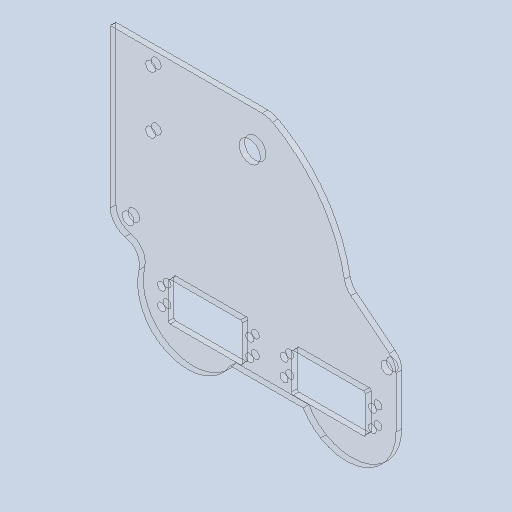
# Autodesk Inventor part: Intake Sides V4_servo
Saved by Autodesk Inventor 2022 (Build 260153000, 153)
## iProperties
Created: 2022-10-16
Part Number: Intake Sides V4_servo
Material: Polycarbonate, Clear
Document SubType Name: Modeling
Designer: matt
Density: 1.2 g/cm^3
Appearance: Polycarbonate - Clear
Mass: 60.255 g
Surface Area: 348.282 cm^2
Volume: 50.2125 cm^3
Author: matt
Autodesk Inventor part; units mm, degrees
ref_plane "YZ Plane" through (0, 0, 0) normal (1, 0, 0) x (0, 1, 0)
ref_plane "XZ Plane" through (0, 0, 0) normal (0, 1, 0) x (-1, 0, 0)
ref_plane "XY Plane" through (0, 0, 0) normal (0, 0, 1) x (1, 0, 0)
sketch "Sketch1" plane through (0, 0, 0) normal (0, 0, 1) x (1, 0, 0)
  arc A0 (16.121808, -110.692366) -> (67.383886, -131.656361) centre (43.321682, -117.338179) ccw
  line L0 (67.383886, -131.656361) -> (108.159478, -131.656361)
  arc A1 (108.159478, -131.656361) -> (139.594615, -90.326332) centre (132.221682, -117.338179) ccw
  arc A2 (132.227805, -80.679244) -> (139.594615, -90.326332) centre (142.227805, -80.679244) ccw
  line L1 (132.227805, -80.679244) -> (132.227805, -71.827)
  arc A3 (132.227805, -71.827) -> (90.658044, -1.487819) centre (51.933317, -71.827) ccw
  arc A4 (90.658044, -1.487819) -> (84.870639, 0) centre (84.870639, -12) ccw
  line L2 (84.870639, 0) -> (0, 0)
  line L3 (0, 0) -> (0, -88.644145)
  arc A5 (0, -88.644145) -> (8.203784, -98.481503) centre (10, -88.644145) ccw
  arc A6 (16.121808, -110.692366) -> (8.203784, -98.481503) centre (6.407567, -108.318861) ccw
  circle A7 centre (121.188208, -82.443861) radius 3.3
  arc A8 (145.794404, -114.286904) -> (148.095336, -110.420107) centre (146.970651, -112.368846) ccw
  circle A9 centre (97.470651, -122.368861) radius 2.25
  circle A10 centre (97.470651, -112.368852) radius 2.25
  circle A11 centre (78.175839, -122.368861) radius 2.25
  arc A12 (145.794404, -124.286918) -> (148.095336, -120.420122) centre (146.970651, -122.368861) ccw
  circle A13 centre (22.617078, -8.511936) radius 2.8
  circle A14 centre (22.617078, -40.511936) radius 2.8
  circle A15 centre (28.675839, -122.368861) radius 2.25
  circle A16 centre (28.675837, -112.368861) radius 2.25
  circle A17 centre (78.175837, -112.368855) radius 2.25
  circle A18 centre (10, -88.644145) radius 3.3
  line L4 (73.060526, -128.291526) -> (33.526976, -128.291526)
  arc A19 (32.526976, -127.291526) -> (33.526976, -128.291526) centre (33.526976, -127.291526) ccw
  line L5 (32.526976, -127.291526) -> (32.526973, -107.491526)
  arc A20 (33.526973, -106.491526) -> (32.526973, -107.491526) centre (33.526973, -107.491526) ccw
  line L6 (33.526973, -106.491526) -> (73.060526, -106.491526)
  arc A21 (74.060526, -107.491526) -> (73.060526, -106.491526) centre (73.060526, -107.491526) ccw
  line L7 (74.060526, -107.491526) -> (74.060526, -127.291526)
  arc A22 (73.060526, -128.291526) -> (74.060526, -127.291526) centre (73.060526, -127.291526) ccw
  line L8 (142.119512, -128.291526) -> (102.585962, -128.291526)
  arc A23 (101.585962, -127.291526) -> (102.585962, -128.291526) centre (102.585962, -127.291526) ccw
  line L9 (101.585962, -127.291526) -> (101.585962, -107.491526)
  arc A24 (102.585962, -106.491526) -> (101.585962, -107.491526) centre (102.585962, -107.491526) ccw
  line L10 (102.585962, -106.491526) -> (142.119515, -106.491526)
  arc A25 (143.119515, -107.491526) -> (142.119515, -106.491526) centre (142.119515, -107.491526) ccw
  line L11 (143.119515, -107.491526) -> (143.119512, -127.291526)
  arc A26 (142.119512, -128.291526) -> (143.119512, -127.291526) centre (142.119512, -127.291526) ccw
  circle A27 centre (146.970651, -112.368846) radius 2.25
  circle A28 centre (146.970651, -122.368861) radius 2.25
  line L12 (28.675837, -112.368861) -> (146.970651, -112.368846) construction
  line L13 (28.675839, -122.368861) -> (146.970651, -122.368861) construction
  circle A29 centre (43.373245, -117.368861) radius 6
  line L14 (67.43545, -131.687043) -> (108.211041, -131.687043)
  arc A30 (108.211041, -131.687043) -> (160.273251, -117.36885) centre (132.273245, -117.36885) ccw
  line L15 (160.273251, -117.36885) -> (160.273251, -88.823719)
  arc A31 (160.273251, -88.823719) -> (156.504028, -81.00212) centre (150.273251, -88.823719) ccw
  line L16 (156.504028, -81.00212) -> (134.936633, -63.821281)
  arc A32 (131.322196, -57.752321) -> (134.936633, -63.821281) centre (141.167411, -55.999682) ccw
  arc A33 (131.322196, -57.752321) -> (90.995274, -1.485865) centre (52.270547, -71.825046) ccw
  arc A34 (90.995274, -1.485865) -> (85.207869, 0.001954) centre (85.207869, -11.998046) ccw
  line L17 (85.207869, 0.001954) -> (0.051563, 0.001954)
  line L18 (0.051563, 0.001954) -> (0.051563, -88.674827)
  arc A35 (0.051563, -88.674827) -> (8.255347, -98.512185) centre (10.051563, -88.674827) ccw
  arc A36 (16.173371, -110.723048) -> (8.255347, -98.512185) centre (6.45913, -108.349543) ccw
  arc A37 (16.173371, -110.723048) -> (67.43545, -131.687043) centre (43.373245, -117.368861) ccw
  circle A38 centre (22.617078, -40.511936) radius 2.8
  circle A39 centre (22.617078, -8.511936) radius 2.8
  circle A40 centre (155.051563, -88.644145) radius 3.3
  circle A41 centre (10.051563, -88.644145) radius 3.3
  circle A42 centre (132.273245, -117.36885) radius 6
  circle A43 centre (78.175837, -21.998046) radius 3.25
  circle A44 centre (78.175837, -21.998046) radius 6
  point P0 (58.854578, -117.368861)
  point P1 (148.095336, -110.420107)
  point P2 (117.931008, -141.41673)
  point P3 (0.051563, 0)
  dimension "d2" = 49.5
  dimension "d3" = 49.5
  dimension "d4" = 49.5
  dimension "d5" = 49.5
  dimension "d6" = 10
  dimension "d7" = 12
  dimension "d8" = 22
  constraints: 34 point on circle, 31 centre point, 28 end point, 4 point on line, 3 coincident, 2 concentric, 1 horizontal, 1 perpendicular
  measures "d2" distance of A17.centre L12.start
  measures "d3" distance of A11.centre L13.start
  measures "d4" distance of L13.end A9.centre
  measures "d5" distance of L12.end A10.centre
  measures "d6" distance of L13.start L12.start
  measures "d7" diameter of A44
  measures "d8" distance from line of A44.centre L17
sketch "Sketch1 outline for Extrusion1" plane through (0, 0, 0) normal (0, 0, 1) x (1, 0, 0)
  line L0 (85.207869, 0.001954) -> (0, 0)
  line L1 (0, 0) -> (0, -88.644145)
  arc A0 (0, -88.644145) -> (8.203784, -98.481503) centre (10, -88.644145) ccw
  arc A1 (8.203784, -98.481503) -> (16.121808, -110.692366) centre (6.407567, -108.318861) cw
  arc A2 (16.121808, -110.692366) -> (67.383886, -131.656361) centre (43.321682, -117.338179) ccw
  line L2 (67.383886, -131.656361) -> (108.159478, -131.656361)
  arc A3 (108.159478, -131.656361) -> (117.931008, -141.41673) centre (132.221682, -117.338179) ccw
  arc A4 (117.931008, -141.41673) -> (160.273251, -117.36885) centre (132.273245, -117.36885) ccw
  line L3 (160.273251, -117.36885) -> (160.273251, -88.823719)
  arc A5 (160.273251, -88.823719) -> (156.504028, -81.00212) centre (150.273251, -88.823719) ccw
  line L4 (156.504028, -81.00212) -> (134.936633, -63.821281)
  arc A6 (134.936633, -63.821281) -> (131.322196, -57.752321) centre (141.167411, -55.999682) cw
  arc A7 (131.322196, -57.752321) -> (90.995274, -1.485865) centre (52.270547, -71.825046) ccw
  arc A8 (90.995274, -1.485865) -> (85.207869, 0.001954) centre (85.207869, -11.998046) ccw
  circle A9 centre (155.051563, -88.644145) radius 3.3
  circle A10 centre (78.175837, -21.998046) radius 6
  circle A11 centre (22.617078, -8.511936) radius 2.8
  circle A12 centre (22.617078, -40.511936) radius 2.8
  circle A13 centre (146.970651, -112.368846) radius 2.25
  circle A14 centre (28.675839, -122.368861) radius 2.25
  circle A15 centre (28.675837, -112.368861) radius 2.25
  line L5 (74.060526, -107.491526) -> (74.060526, -127.291526)
  arc A16 (74.060526, -127.291526) -> (73.060526, -128.291526) centre (73.060526, -127.291526) cw
  line L6 (73.060526, -128.291526) -> (33.526976, -128.291526)
  arc A17 (33.526976, -128.291526) -> (32.526976, -127.291526) centre (33.526976, -127.291526) cw
  line L7 (32.526976, -127.291526) -> (32.526973, -107.491526)
  arc A18 (32.526973, -107.491526) -> (33.526973, -106.491526) centre (33.526973, -107.491526) cw
  line L8 (33.526973, -106.491526) -> (73.060526, -106.491526)
  arc A19 (73.060526, -106.491526) -> (74.060526, -107.491526) centre (73.060526, -107.491526) cw
  circle A20 centre (10, -88.644145) radius 3.3
  circle A21 centre (78.175839, -122.368861) radius 2.25
  circle A22 centre (97.470651, -122.368861) radius 2.25
  circle A23 centre (78.175837, -112.368855) radius 2.25
  circle A24 centre (97.470651, -112.368852) radius 2.25
  line L9 (102.585962, -106.491526) -> (142.119515, -106.491526)
  arc A25 (142.119515, -106.491526) -> (143.119515, -107.491526) centre (142.119515, -107.491526) cw
  line L10 (143.119515, -107.491526) -> (143.119512, -127.291526)
  arc A26 (143.119512, -127.291526) -> (142.119512, -128.291526) centre (142.119512, -127.291526) cw
  line L11 (142.119512, -128.291526) -> (102.585962, -128.291526)
  arc A27 (102.585962, -128.291526) -> (101.585962, -127.291526) centre (102.585962, -127.291526) cw
  line L12 (101.585962, -127.291526) -> (101.585962, -107.491526)
  arc A28 (101.585962, -107.491526) -> (102.585962, -106.491526) centre (102.585962, -107.491526) cw
  circle A29 centre (146.970651, -122.368861) radius 2.25
extrude "Extrusion1" add sketch "Sketch1 outline for Extrusion1" along normal blind 3.175
body "Solid1"
